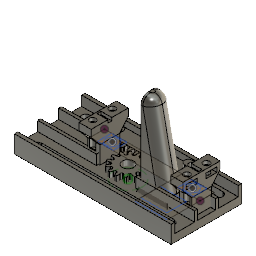
RP_Gripper_MK4_v10 (Autodesk Fusion 360 design; units mm, degrees)
description: Spur Gear; Module: 1.072000; Num Teeth: 14; Pressure Angle: 14.500000; Backlash: 0.15 mm
description: Spur Gear; Module: 1.020000; Num Teeth: 14; Pressure Angle: 14.500000; Backlash: 0.15 mm
Autodesk Fusion 360 part; units mm, degrees
sketch "Sketch1" plane through (0, 0, 0) normal (0, 0, 1) x (1, 0, 0) in component "Old Spur (14 teeth)"
  circle A0 centre (0, 0) radius 6.1668
  circle A1 centre (0, 0) radius 1.6
extrude "Extrude1" add sketch "Sketch1" along normal blind 6.5 makes body 1 in component "Old Spur (14 teeth)"
sketch "Sketch2" plane through (0, 0, 0) normal (0, 0, 1) x (1, 0, 0) in component "Old Spur (14 teeth)"
  spline S0 degree 5 poles (7.2189, -0.8174) (7.2227, -0.8178) (7.2303, -0.8185) (7.2417, -0.8194) (7.257, -0.8199) (7.2761, -0.8197) (7.2953, -0.819) (7.3145, -0.8178) (7.3337, -0.8165) (7.353, -0.815) (7.3723, -0.8134) (7.3915, -0.8117) (7.4108, -0.8096) (7.4302, -0.8073) (7.4495, -0.8047) (7.4688, -0.8019) (7.4882, -0.7988) (7.5075, -0.7955) (7.5269, -0.7921) (7.5463, -0.7884) (7.5657, -0.7847) (7.585, -0.7807) (7.6044, -0.7766) (7.6238, -0.7723) (7.6432, -0.7679) (7.6626, -0.7632) (7.682, -0.7584) (7.7014, -0.7534) (7.7208, -0.7483) (7.7402, -0.743) (7.7596, -0.7376) (7.779, -0.7321) (7.7984, -0.7264) (7.8177, -0.7205) (7.8371, -0.7145) (7.8565, -0.7084) (7.8759, -0.7021) (7.8953, -0.6956) (7.9146, -0.6891) (7.934, -0.6824) (7.9533, -0.6756) (7.9727, -0.6686) (7.992, -0.6615) (8.0114, -0.6543) (8.0307, -0.6469) (8.05, -0.6394) (8.0693, -0.6318) (8.0886, -0.6241) (8.1079, -0.6162) (8.1272, -0.6082) (8.1465, -0.6001) (8.1657, -0.5919) (8.185, -0.5835) (8.2042, -0.575) (8.2234, -0.5664) (8.2427, -0.5577) (8.2619, -0.5489) (8.281, -0.5399) (8.3002, -0.5309) (8.3194, -0.5217) (8.3385, -0.5124) (8.3577, -0.5029) (8.3768, -0.4934) (8.3959, -0.4837) (8.415, -0.474) (8.434, -0.4641) (8.4531, -0.4541) (8.4721, -0.444) (8.4911, -0.4338) (8.5101, -0.4235) (8.5291, -0.413) (8.5443, -0.4046) (8.5557, -0.3982) (8.5633, -0.394) (8.567, -0.3918) knots 0 0 0 0 0 0 0.01428571 0.02857143 0.04285714 0.05714286 0.07142857 0.08571429 0.1 0.11428571 0.12857143 0.14285714 0.15714286 0.17142857 0.18571429 0.2 0.21428571 0.22857143 0.24285714 0.25714286 0.27142857 0.28571429 0.3 0.31428571 0.32857143 0.34285714 0.35714286 0.37142857 0.38571429 0.4 0.41428571 0.42857143 0.44285714 0.45714286 0.47142857 0.48571429 0.5 0.51428571 0.52857143 0.54285714 0.55714286 0.57142857 0.58571429 0.6 0.61428571 0.62857143 0.64285714 0.65714286 0.67142857 0.68571429 0.7 0.71428571 0.72857143 0.74285714 0.75714286 0.77142857 0.78571429 0.8 0.81428571 0.82857143 0.84285714 0.85714286 0.87142857 0.88571429 0.9 0.91428571 0.92857143 0.94285714 0.95714286 0.97142857 0.98571429 1 1 1 1 1 1
  spline S1 degree 5 poles (7.2189, 0.8174) (7.2227, 0.8178) (7.2303, 0.8185) (7.2417, 0.8194) (7.257, 0.8199) (7.2761, 0.8197) (7.2953, 0.819) (7.3145, 0.8178) (7.3337, 0.8165) (7.353, 0.815) (7.3723, 0.8134) (7.3915, 0.8117) (7.4108, 0.8096) (7.4302, 0.8073) (7.4495, 0.8047) (7.4688, 0.8019) (7.4882, 0.7988) (7.5075, 0.7955) (7.5269, 0.7921) (7.5463, 0.7884) (7.5657, 0.7847) (7.585, 0.7807) (7.6044, 0.7766) (7.6238, 0.7723) (7.6432, 0.7679) (7.6626, 0.7632) (7.682, 0.7584) (7.7014, 0.7534) (7.7208, 0.7483) (7.7402, 0.743) (7.7596, 0.7376) (7.779, 0.7321) (7.7984, 0.7264) (7.8177, 0.7205) (7.8371, 0.7145) (7.8565, 0.7084) (7.8759, 0.7021) (7.8953, 0.6956) (7.9146, 0.6891) (7.934, 0.6824) (7.9533, 0.6756) (7.9727, 0.6686) (7.992, 0.6615) (8.0114, 0.6543) (8.0307, 0.6469) (8.05, 0.6394) (8.0693, 0.6318) (8.0886, 0.6241) (8.1079, 0.6162) (8.1272, 0.6082) (8.1465, 0.6001) (8.1657, 0.5919) (8.185, 0.5835) (8.2042, 0.575) (8.2234, 0.5664) (8.2427, 0.5577) (8.2619, 0.5489) (8.281, 0.5399) (8.3002, 0.5309) (8.3194, 0.5217) (8.3385, 0.5124) (8.3577, 0.5029) (8.3768, 0.4934) (8.3959, 0.4837) (8.415, 0.474) (8.434, 0.4641) (8.4531, 0.4541) (8.4721, 0.444) (8.4911, 0.4338) (8.5101, 0.4235) (8.5291, 0.413) (8.5443, 0.4046) (8.5557, 0.3982) (8.5633, 0.394) (8.567, 0.3918) knots 0 0 0 0 0 0 0.01428571 0.02857143 0.04285714 0.05714286 0.07142857 0.08571429 0.1 0.11428571 0.12857143 0.14285714 0.15714286 0.17142857 0.18571429 0.2 0.21428571 0.22857143 0.24285714 0.25714286 0.27142857 0.28571429 0.3 0.31428571 0.32857143 0.34285714 0.35714286 0.37142857 0.38571429 0.4 0.41428571 0.42857143 0.44285714 0.45714286 0.47142857 0.48571429 0.5 0.51428571 0.52857143 0.54285714 0.55714286 0.57142857 0.58571429 0.6 0.61428571 0.62857143 0.64285714 0.65714286 0.67142857 0.68571429 0.7 0.71428571 0.72857143 0.74285714 0.75714286 0.77142857 0.78571429 0.8 0.81428571 0.82857143 0.84285714 0.85714286 0.87142857 0.88571429 0.9 0.91428571 0.92857143 0.94285714 0.95714286 0.97142857 0.98571429 1 1 1 1 1 1
  arc A0 (8.567, -0.3918) -> (8.567, 0.3918) centre (0, 0) ccw
  line L0 (6.1177, -0.6938) -> (7.2189, -0.8174)
  line L1 (6.1177, 0.6938) -> (7.2189, 0.8174)
  line L2 (6.1177, -0.6938) -> (6.1177, 0.6938)
  point P0 (7.313, -0.8179)
  point P1 (7.4081, -0.8099)
  point P2 (7.5038, -0.7961)
  point P3 (7.5999, -0.7776)
  point P4 (7.6963, -0.7547)
  point P5 (7.7929, -0.7279)
  point P6 (7.8897, -0.6975)
  point P7 (7.9866, -0.6635)
  point P8 (8.0836, -0.6261)
  point P9 (8.1805, -0.5854)
  point P10 (8.2774, -0.5416)
  point P11 (8.3741, -0.4947)
  point P12 (8.4707, -0.4448)
  point P13 (7.313, 0.8179)
  point P14 (7.4081, 0.8099)
  point P15 (7.5038, 0.7961)
  point P16 (7.5999, 0.7776)
  point P17 (7.6963, 0.7547)
  point P18 (7.7929, 0.7279)
  point P19 (7.8897, 0.6975)
  point P20 (7.9866, 0.6635)
  point P21 (8.0836, 0.6261)
  point P22 (8.1805, 0.5854)
  point P23 (8.2774, 0.5416)
  point P24 (8.3741, 0.4947)
  point P25 (8.4707, 0.4448)
extrude "Extrude2" add sketch "Sketch2" along normal blind 6.5 bodies 1 in component "Old Spur (14 teeth)"
fillet "Fillet1" radius 0.6 2 edges at (6.1275, -0.6949, 3.25) (6.1275, 0.6949, 3.25) on bodies 1 in component "Old Spur (14 teeth)"
pattern_circular "C-Pattern1" count 14 over 360 about axis through (0, 0, 0) along (0, 0, 1) of "Extrude2", "Fillet1" in component "Old Spur (14 teeth)"
sketch "Sketch3" plane through (0, 0, 0) normal (0, 0, 1) x (1, 0, 0) in component "Old Spur (14 teeth)"
  circle A0 centre (0, 0) radius 7.504 construction
sketch "Sketch1 (2)" plane through (0, 0, 0) normal (0, 0, 1) x (1, 0, 0) in component "Rack"
  line L0 (-30, 8.75) -> (30, 8.75)
  line L1 (30, 8.75) -> (30, 12.75)
  line L2 (30, 12.75) -> (-30, 12.75)
  line L3 (-30, 12.75) -> (-30, 8.75)
  line L4 (0.1675, 6.2955) -> (-0.167, 6.2955)
  line L5 (-0.6525, 6.781) -> (-0.6525, 7.2573)
  line L6 (-0.6525, 9.4955) -> (0.6525, 9.4955)
  line L7 (0.6525, 9.4955) -> (0.6525, 6.7805)
  line L8 (0.6525, 6.2955) -> (-0.6525, 9.4955) construction
  line L9 (-0.6525, 6.2955) -> (0.6525, 9.4955) construction
  arc A0 (-0.6525, 6.781) -> (-0.167, 6.2955) centre (-0.167, 6.781) ccw
  arc A1 (0.1675, 6.2955) -> (0.6525, 6.7805) centre (0.1675, 6.7805) ccw
  arc A2 (-0.6724, 7.5148) -> (-1.0506, 8.75) centre (-5.1412, 6.8218) ccw
  arc A3 (-0.6525, 7.2573) -> (-0.6724, 7.5148) centre (-2.3332, 7.2573) ccw
  line L10 (0, 10) -> (0, 5.7453) construction
  arc A4 (1.0506, 8.75) -> (0.6724, 7.5148) centre (5.1412, 6.8218) ccw
  arc A5 (0.6724, 7.5148) -> (0.6525, 7.2573) centre (2.3332, 7.2573) ccw
  point P0 (0, 7.8955)
  dimension "d8" = 3.2
  dimension "d9" = 1.305
  dimension "d10" = 0.4855
  dimension "d11" = 0.485
  dimension "d12" = 1.6807
  constraint horizontal L0
  constraint vertical L1
  constraint horizontal L2
  constraint vertical L3
  constraint perpendicular L4 L5
  constraint parallel L4 L6
  constraint parallel L5 L7
  constraint horizontal L4
  constraint coincident L8 P0
  constraint coincident L9 P0
  constraint coincident L9.start L4
  constraint coincident L9.start L5
  constraint tangent L4 A0
  constraint tangent L5 A0
  constraint tangent L7 A1
  constraint tangent L4 A1
  constraint coincident L0 A2.end
  constraint coincident L6.start L5
  constraint tangent L5 A3
  constraint tangent A2 A3
  constraint perpendicular L6 L10
  constraint symmetric A2.end L10 A4.start
  constraint symmetric A2 L10 A4
  constraint symmetric L5.end L10 A5.end
  constraint symmetric A2.start L10 A4.end
  constraint symmetric A3 L10 A5
  measures "d8" distance of L9.start L6.start
  measures "d9" distance of L6.start L6.end
  measures "d10" radius of A0
  measures "d11" radius of A1
  measures "d12" radius of A3
copy_body "CopyPasteBodies1" bodies 1 makes body 2 in component "Old Spur (14 teeth)"
move_body "Move1" bodies 2 to x (0.975535, 0.219846, 0) y (-0.219846, 0.975535, 0) z (0, 0, 1) at (0, 0, 0) in component "Old Spur (14 teeth)"
extrude "Extrude1'" add sketch "Sketch1 (2)" along normal blind 6 separate body contours L0 L4 L5 L7 A0 A1 A2 A3 | L0 L7 A4 A5 makes body 3 in component "Rack"
move_body "Move2" bodies 2 to x (1, 0, 0) y (0, 1, 0) z (0, 0, 1) at (-1.6805, 0, 0) in component "Old Spur (14 teeth)"
copy_body "CopyPasteBodies1'" bodies 3 makes body 4 in component "Rack"
move_body "Move1'" bodies 4 to x (1, 0, 0) y (0, 1, 0) z (0, 0, 1) at (-3.31, 0, 0) in component "Rack"
copy_body "CopyPasteBodies2" bodies 4 makes body 5 in component "Rack"
move_body "Move2'" bodies 5 to x (1, 0, 0) y (0, 1, 0) z (0, 0, 1) at (-3.31, 0, 0) in component "Rack"
copy_body "CopyPasteBodies3" bodies 5 makes body 6 in component "Rack"
move_body "Move3" bodies 6 to x (1, 0, 0) y (0, 1, 0) z (0, 0, 1) at (-3.31, 0, 0) in component "Rack"
copy_body "CopyPasteBodies4" bodies 6 makes body 7 in component "Rack"
move_body "Move4" bodies 7 to x (1, 0, 0) y (0, 1, 0) z (0, 0, 1) at (-3.31, 0, 0) in component "Rack"
copy_body "CopyPasteBodies5" bodies 7 makes body 8 in component "Rack"
move_body "Move5" bodies 8 to x (1, 0, 0) y (0, 1, 0) z (0, 0, 1) at (-3.31, 0, 0) in component "Rack"
copy_body "CopyPasteBodies6" bodies 8 makes body 9 in component "Rack"
move_body "Move6" bodies 9 to x (1, 0, 0) y (0, 1, 0) z (0, 0, 1) at (-3.31, 0, 0) in component "Rack"
copy_body "CopyPasteBodies7" bodies 9 makes body 10 in component "Rack"
move_body "Move7" bodies 10 to x (1, 0, 0) y (0, 1, 0) z (0, 0, 1) at (-3.31, 0, 0) in component "Rack"
copy_body "CopyPasteBodies8" bodies 10 makes body 11 in component "Rack"
move_body "Move8" bodies 11 to x (1, 0, 0) y (0, 1, 0) z (0, 0, 1) at (-3.31, 0, 0) in component "Rack"
copy_body "CopyPasteBodies9" bodies 3 makes body 12 in component "Rack"
move_body "Move9" bodies 12 to x (1, 0, 0) y (0, 1, 0) z (0, 0, 1) at (3.31, 0, 0) in component "Rack"
copy_body "CopyPasteBodies10" bodies 12 makes body 13 in component "Rack"
move_body "Move10" bodies 13 to x (1, 0, 0) y (0, 1, 0) z (0, 0, 1) at (3.31, 0, 0) in component "Rack"
copy_body "CopyPasteBodies11" bodies 13 makes body 14 in component "Rack"
move_body "Move11" bodies 14 to x (1, 0, 0) y (0, 1, 0) z (0, 0, 1) at (3.31, 0, 0) in component "Rack"
copy_body "CopyPasteBodies12" bodies 14 makes body 15 in component "Rack"
move_body "Move12" bodies 15 to x (1, 0, 0) y (0, 1, 0) z (0, 0, 1) at (3.31, 0, 0) in component "Rack"
copy_body "CopyPasteBodies13" bodies 15 makes body 16 in component "Rack"
move_body "Move13" bodies 16 to x (1, 0, 0) y (0, 1, 0) z (0, 0, 1) at (3.31, 0, 0) in component "Rack"
copy_body "CopyPasteBodies14" bodies 16 makes body 17 in component "Rack"
move_body "Move14" bodies 17 to x (1, 0, 0) y (0, 1, 0) z (0, 0, 1) at (3.31, 0, 0) in component "Rack"
copy_body "CopyPasteBodies15" bodies 17 makes body 18 in component "Rack"
move_body "Move15" bodies 18 to x (1, 0, 0) y (0, 1, 0) z (0, 0, 1) at (3.31, 0, 0) in component "Rack"
copy_body "CopyPasteBodies16" bodies 18 makes body 19 in component "Rack"
move_body "Move16" bodies 19 to x (1, 0, 0) y (0, 1, 0) z (0, 0, 1) at (3.31, 0, 0) in component "Rack"
sketch "Sketch2 (2)" plane through (0, 0, 0) normal (0, 0, 1) x (1, 0, 0) in component "Rack"
  line L0 (28, 16) -> (-28, 16)
  line L1 (-28, 16) -> (-28, 8.75)
  line L2 (-28, 8.75) -> (28, 8.75)
  line L3 (28, 8.75) -> (28, 16)
  dimension "d15" = 56
  dimension "d16" = 7.25
  constraint horizontal L0
  constraint vertical L1
  constraint horizontal L2
  constraint vertical L3
  measures "d15" distance of L0.start L0.end
  measures "d16" distance of L0.start L2.end
extrude "Extrude2'" add sketch "Sketch2 (2)" along normal blind 6 separate body makes body 20 in component "Rack"
sketch "Sketch1 (3)" plane through (0, 0, 0) normal (0, 0, 1) x (1, 0, 0) in component "Base"
  line L0 (40, 18) -> (-40, 18)
  line L1 (-40, 18) -> (-40, -18)
  line L2 (-40, -18) -> (40, -18)
  line L3 (40, -18) -> (40, 18)
  line L4 (-40, 18) -> (40, 18)
  line L5 (40, 18) -> (40, 16.2)
  line L6 (40, 16.2) -> (-40, 16.2)
  line L7 (-40, 16.2) -> (-40, 18)
  line L8 (40, 4.6) -> (10, 4.6)
  line L9 (10, 4.6) -> (10, 6.1)
  line L10 (10, 6.1) -> (40, 6.1)
  line L11 (40, 6.1) -> (40, 4.6)
  line L12 (-40, 4.6) -> (-10, 4.6)
  line L13 (-10, 4.6) -> (-10, 6.1)
  line L14 (-10, 6.1) -> (-40, 6.1)
  line L15 (-40, 6.1) -> (-40, 4.6)
  line L16 (-40, -18) -> (40, -18)
  line L17 (40, -18) -> (40, -16.2)
  line L18 (40, -16.2) -> (-40, -16.2)
  line L19 (-40, -16.2) -> (-40, -18)
  line L20 (40, -4.6) -> (10, -4.6)
  line L21 (10, -4.6) -> (10, -6.1)
  line L22 (10, -6.1) -> (40, -6.1)
  line L23 (40, -6.1) -> (40, -4.6)
  line L24 (-40, -4.6) -> (-10, -4.6)
  line L25 (-10, -4.6) -> (-10, -6.1)
  line L26 (-10, -6.1) -> (-40, -6.1)
  line L27 (-40, -6.1) -> (-40, -4.6)
  line L28 (45.5245, 12.375) -> (-50, 12.375) construction
  line L29 (33.9, 14.475) -> (-33.9, 14.475)
  line L30 (-36, 12.375) -> (-36, 12.375)
  line L31 (-33.9, 10.275) -> (33.9, 10.275)
  line L32 (36, 12.375) -> (36, 12.375)
  arc A0 (33.9, 10.275) -> (36, 12.375) centre (33.9, 12.375) ccw
  arc A1 (36, 12.375) -> (33.9, 14.475) centre (33.9, 12.375) ccw
  arc A2 (-33.9, 14.475) -> (-36, 12.375) centre (-33.9, 12.375) ccw
  arc A3 (-36, 12.375) -> (-33.9, 10.275) centre (-33.9, 12.375) ccw
  line L33 (45, 0) -> (-44, 0) construction
  arc A4 (-36, -12.375) -> (-33.9, -14.475) centre (-33.9, -12.375) ccw
  arc A5 (-33.9, -10.275) -> (-36, -12.375) centre (-33.9, -12.375) ccw
  line L34 (-33.9, -10.275) -> (33.9, -10.275)
  line L35 (33.9, -14.475) -> (-33.9, -14.475)
  arc A6 (36, -12.375) -> (33.9, -10.275) centre (33.9, -12.375) ccw
  arc A7 (33.9, -14.475) -> (36, -12.375) centre (33.9, -12.375) ccw
  point P0 (36, 14.475)
  point P1 (36, 10.275)
  dimension "d19" = 1.8
  dimension "d20" = 80
  dimension "d21" = 30
  dimension "d22" = 1.5
  dimension "d23" = 10.1
  dimension "d24" = 30
  dimension "d25" = 1.5
  dimension "d26" = 10.1
  dimension "d27" = 80
  dimension "d28" = 1.8
  dimension "d29" = 30
  dimension "d30" = 1.5
  dimension "d31" = 10.1
  dimension "d32" = 30
  dimension "d33" = 1.5
  dimension "d34" = 10.1
  dimension "d35" = 4.2
  dimension "d36" = 2.1
  dimension "d37" = 2.1
  dimension "d38" = 2.1
  dimension "d39" = 2.1
  dimension "d40" = 2.1
  constraint horizontal L0
  constraint vertical L1
  constraint horizontal L2
  constraint vertical L3
  constraint horizontal L4
  constraint vertical L5
  constraint horizontal L6
  constraint vertical L7
  constraint horizontal L8
  constraint vertical L9
  constraint horizontal L10
  constraint vertical L11
  constraint coincident L3 L8.start
  constraint horizontal L12
  constraint vertical L13
  constraint horizontal L14
  constraint vertical L15
  constraint coincident L1 L12.start
  constraint horizontal L16
  constraint vertical L17
  constraint horizontal L18
  constraint vertical L19
  constraint horizontal L20
  constraint vertical L21
  constraint horizontal L22
  constraint vertical L23
  constraint coincident L3 L20.start
  constraint horizontal L24
  constraint vertical L25
  constraint horizontal L26
  constraint vertical L27
  constraint coincident L1 L24.start
  constraint perpendicular L3 L28
  constraint horizontal L29
  constraint horizontal L31
  constraint coincident P1 L31
  constraint tangent L31 A0
  constraint coincident P0 L29
  constraint coincident P0 L32
  constraint tangent L29 A1
  constraint tangent L29 A2
  constraint tangent L31 A3
  constraint perpendicular L3 L33
  constraint symmetric L31.end L33 L34.end
  constraint symmetric L32.start L33 A6.start
  constraint symmetric A0 L33 A6
  constraint symmetric L29.start L33 L35.start
  constraint symmetric A1 L33 A7
  constraint symmetric L29.end L33 A4.end
  constraint symmetric L30.start L33 A4.start
  constraint symmetric A2 L33 A4
  constraint symmetric L31.start L33 A5.start
  constraint symmetric A3 L33 A5
  measures "d19" distance of L0.end L6.end
  measures "d20" distance of L0.end L0.start
  measures "d21" distance of L8.start L8.end
  measures "d22" distance of L8.start L10.end
  measures "d23" distance of L6 L10
  measures "d24" distance of L12.start L12.end
  measures "d25" distance of L12.start L14.end
  measures "d26" distance of L6 L14
  measures "d27" distance of L1.end L2.end
  measures "d28" distance of L1.end L18.end
  measures "d29" distance of L20.start L20.end
  measures "d30" distance of L20.start L22.end
  measures "d31" distance of L18 L22
  measures "d32" distance of L24.start L24.end
  measures "d33" distance of L24.start L26.end
  measures "d34" distance of L18 L26
  measures "d35" distance of P0 P1
  measures "d36" distance of L28 L29
  measures "d37" radius of A0
  measures "d38" radius of A1
  measures "d39" radius of A2
  measures "d40" radius of A3
extrude "Extrude1''" add sketch "Sketch1 (3)" along normal blind 4 separate body makes body 21 in component "Base"
extrude "Extrude2''" add sketch "Sketch1 (3)" along normal blind 9 contours L0 L1 L3 L4 L5 L6 L7 | L3 L8 L9 L10 L11 | L1 L12 L13 L14 L15 | L3 L20 L21 L22 L23 | L1 L24 L25 L26 L27 | L1 L2 L3 L16 L17 L18 L19 bodies 21 in component "Base"
box "BoxPrimitive1" add length 10 width 6.25 height 9 placed x (0, -1, 0) y (1, 0, 0) z (0, 0, 1) at (-15.25, 5, 4) separate body makes body 22 in component "Base"
box "BoxPrimitive2" add length 19 width 6.25 height 9 placed x (0, -1, 0) y (1, 0, 0) z (0, 0, 1) at (-15.25, 8.9473, 13) separate body makes body 23 in component "Base"
move_body "Move1''" bodies 23 to x (1, 0, 0) y (0, 1, 0) z (0, 0, 1) at (0, 0, 15.6817) in component "Base"
move_body "Align1" bodies 23 to x (1, 0, 0) y (0, 1, 0) z (0, 0, 1) at (0, 0.5527, -15.6817) in component "Base"
chamfer "Chamfer1" distance 4.5 angle 50 2 edges at (-12.125, -9.5, 13) (-12.125, 9.5, 13) measured on face at (-11.0833, 3.1667, 13) measured on face at (-11.0833, 3.1667, 13) on bodies 23 in component "Base"
sketch "Sketch4" plane through (0, 0, 22) normal (0, 0, 1) x (-1, 0, 0) in component "Base"
  line L0 (15.25, 9.5) -> (9, 9.5)
  line L1 (9, 9.5) -> (9, -9.5)
  line L2 (9, -9.5) -> (15.25, -9.5)
  line L3 (15.25, -9.5) -> (15.25, 9.5)
  circle A0 centre (12.75, -5) radius 1.6
  circle A1 centre (12.75, 5) radius 1.6
  line L4 (9, 1) -> (14.5, 1)
  line L5 (14.5, 1) -> (14.5, -1)
  line L6 (14.5, -1) -> (9, -1)
  line L7 (9, -1) -> (9, 1)
  dimension "d57" = 3.2
  dimension "d58" = 4.5
  dimension "d59" = 2.5
  dimension "d60" = 3.2
  dimension "d61" = 2.5
  dimension "d62" = 10
  dimension "d63" = 5.5
  dimension "d64" = 2
  constraint horizontal L4
  constraint vertical L5
  constraint horizontal L6
  constraint vertical L7
  constraint coincident L1 L4.start
  measures "d57" diameter of A0
  measures "d58" distance of L2 A0.centre
  measures "d59" distance of L3 A0.centre
  measures "d60" diameter of A1
  measures "d61" distance of L3 A1.centre
  measures "d62" vertical distance of A0.centre A1.centre
  measures "d63" distance of L4.start L4.end
  measures "d64" distance of L4.start L6.end
extrude "Extrude3" cut sketch "Sketch4" against normal blind 13 contours A0 | A1 bodies 22 23 in component "Base"
extrude "Extrude4" cut sketch "Sketch4" against normal blind 1.5 contours L1 L4 L5 L6 L7 bodies 23 in component "Base"
sketch "Sketch5" plane through (-15.25, 0, 0) normal (-1, 0, 0) x (0, -1, 0) in component "Base"
  line L0 (-9.5, 18.3629) -> (-5, 13)
  line L1 (-5, 13) -> (5, 13)
  line L2 (5, 13) -> (9.5, 18.3629)
  line L3 (9.5, 18.3629) -> (9.5, 22)
  line L4 (9.5, 22) -> (-9.5, 22)
  line L5 (-9.5, 22) -> (-9.5, 18.3629)
  line L6 (-7.8, 20.25) -> (-2.2, 20.25)
  line L7 (-2.2, 20.25) -> (-2.2, 17.75)
  line L8 (-2.2, 17.75) -> (-7.8, 17.75)
  line L9 (-7.8, 17.75) -> (-7.8, 20.25)
  line L10 (-3.4, 22) -> (-6.6, 22)
  line L11 (0, 23) -> (0, 12) construction
  line L12 (7.8, 17.75) -> (7.8, 20.25)
  line L13 (7.8, 20.25) -> (2.2, 20.25)
  line L14 (2.2, 20.25) -> (2.2, 17.75)
  line L15 (2.2, 17.75) -> (7.8, 17.75)
  dimension "d69" = 5.6
  dimension "d70" = 2.5
  dimension "d71" = 1.7
  dimension "d72" = 1.75
  constraint horizontal L6
  constraint vertical L7
  constraint horizontal L8
  constraint vertical L9
  constraint perpendicular L1 L11
  constraint symmetric L6.start L11 L12.end
  constraint symmetric L6.end L11 L13.end
  constraint symmetric L7.end L11 L14.end
  constraint symmetric L8.end L11 L12.start
  measures "d69" distance of L6.start L6.end
  measures "d70" distance of L6.start L8.end
  measures "d71" distance of L5 L9
  measures "d72" distance of L6 L10
extrude "Extrude5" cut sketch "Sketch5" against normal blind 5.6 contours L6 L7 L8 L9 | L12 L13 L14 L15 bodies 23 in component "Base"
copy_body "CopyPasteBodies1''" bodies 22 23 makes body 24 makes body 25 in component "Base"
move_body "Move2''" bodies 24 25 to x (1, 0, 0) y (0, 1, 0) z (0, 0, 1) at (45, 0, 0) in component "Base"
move_body "Move3'" bodies 25 24 to x (-1, 0, 0) y (0, -1, 0) z (0, 0, 1) at (66.5, 0, 0) in component "Base"
move_body "Move4'" bodies 22 23 to x (1, 0, 0) y (0, 1, 0) z (0, 0, 1) at (-4, 0, 0) in component "Base"
move_body "Move5'" bodies 25 24 to x (1, 0, 0) y (0, 1, 0) z (0, 0, 1) at (-3, 0, 0) in component "Base"
box "BoxPrimitive1'" add length 4 width 48.8 height 4.3 placed x (0, -1, 0) y (1, 0, 0) z (0, 0, 1) at (-28, 16, 6) separate body makes body 26 in component "Rack"
move_body "Move17" bodies 26 to x (1, 0, 0) y (0, 1, 0) z (0, 0, 1) at (3.61, 0, 0) in component "Rack"
move_body "Move18" bodies 26 to x (1, 0, 0) y (0, 1, 0) z (0, 0, 1) at (0, -1.625, 0) in component "Rack"
ref_plane "WorkPlane1" through (-16.39, 12.375, 8.15) normal (-1, 0, 0) x (0, 0, -1) in component "Rack"
split "Split1" by plane through (-16.39, 12.375, 8.15) normal (-1, 0, 0) bodies 26 makes body 27 at (-21.7233, 14.375, 7.4333) in component "Rack"
ref_plane "WorkPlane2" through (16.41, 12.375, 8.15) normal (1, 0, 0) x (0, 0, 1) in component "Rack"
split "Split2" by plane through (16.41, 12.375, 8.15) normal (1, 0, 0) bodies 26 makes body 28 at (19.0767, 14.375, 7.4333) in component "Rack"
delete_body "RemoveBody1" bodies 26 in component "Rack"
sketch "Sketch4 (2)" plane through (0, 0, 10.3) normal (0, 0, 1) x (-1, 0, 0) in component "Rack"
  line L0 (16.39, -10.375) -> (16.39, -14.375)
  line L1 (16.39, -14.375) -> (24.39, -14.375)
  line L2 (24.39, -14.375) -> (24.39, -10.375)
  line L3 (24.39, -10.375) -> (16.39, -10.375)
  circle A0 centre (20.39, -12.375) radius 1.65
  dimension "d83" = 3.3
  dimension "d84" = 2
  dimension "d85" = 4
  measures "d83" diameter of A0
  measures "d84" distance of L1 A0.centre
  measures "d85" distance of L2 A0.centre
sketch "Sketch5 (2)" plane through (0, 0, 10.3) normal (0, 0, 1) x (-1, 0, 0) in component "Rack"
  line L0 (-16.41, -14.375) -> (-16.41, -10.375)
  line L1 (-16.41, -10.375) -> (-24.41, -10.375)
  line L2 (-24.41, -10.375) -> (-24.41, -14.375)
  line L3 (-24.41, -14.375) -> (-16.41, -14.375)
  circle A0 centre (-20.41, -12.375) radius 1.65
  dimension "d86" = 3.3
  dimension "d87" = 4
  dimension "d88" = 2
  measures "d86" diameter of A0
  measures "d87" distance of L2 A0.centre
  measures "d88" distance of L3 A0.centre
fillet "Fillet2" radius 2 4 edges at (24.41, 10.375, 8.15) (16.41, 10.375, 8.15) (24.41, 14.375, 8.15) (16.41, 14.375, 8.15) on bodies 28 in component "Rack"
fillet "Fillet3" radius 2 4 edges at (-16.39, 14.375, 8.15) (-24.39, 14.375, 8.15) (-24.39, 10.375, 8.15) (-16.39, 10.375, 8.15) on bodies 27 in component "Rack"
extrude "Extrude3'" cut sketch "Sketch4 (2)" against normal blind 21.743 contours A0 bodies 20 27 in component "Rack"
extrude "Extrude4'" cut sketch "Sketch5 (2)" against normal blind 14.123 contours A0 bodies 20 28 in component "Rack"
sketch "Sketch6" plane through (0, 0, 0) normal (0, 0, -1) x (1, 0, 0) in component "Rack"
  circle A0 centre (20.41, -12.375) radius 1.65
  circle A1 centre (-20.39, -12.375) radius 1.65
  line L0 (28, -16) -> (28, -8.75)
  line L1 (28, -8.75) -> (-28, -8.75)
  line L2 (-28, -8.75) -> (-28, -16)
  line L3 (-28, -16) -> (28, -16)
  circle A2 centre (-20.39, -12.375) radius 3.1
  circle A3 centre (20.41, -12.375) radius 3.1
  dimension "d95" = 6.2
  dimension "d96" = 6.2
  constraint concentric A1 A2
  constraint concentric A0 A3
  measures "d95" diameter of A2
  measures "d96" diameter of A3
extrude "Extrude5'" cut sketch "Sketch6" against normal blind 2.8 contours A2 | A3 bodies 20 in component "Rack"
sketch "Sketch1 (4)" plane through (0, 0, 0) normal (0, 0, 1) x (1, 0, 0) in component "Jaw"
  line L0 (-28, 16) -> (28, 16)
  line L1 (28, 16) -> (28, 8.75)
  line L2 (28, 8.75) -> (-28, 8.75)
  line L3 (-28, 8.75) -> (-28, 16)
  line L4 (11.5, 16) -> (28, 16)
  line L5 (28, 16) -> (28, -8)
  line L6 (28, -8) -> (11.5, -8)
  line L7 (11.5, -8) -> (11.5, 16)
  line L8 (11.5, -5) -> (24.8331, -5)
  line L9 (24.8331, -5) -> (24.8331, 5)
  line L10 (24.8331, 5) -> (11.5, 5)
  line L11 (11.5, 5) -> (11.5, -5)
  circle A0 centre (20.4076, 12.375) radius 1.6
  circle A1 centre (-20.3901, 12.3735) radius 1.6
  line L12 (-16.3901, 8.8735) -> (-24.3901, 8.8735)
  line L13 (-24.3901, 8.8735) -> (-24.3901, 15.8735)
  line L14 (-24.3901, 15.8735) -> (-16.3901, 15.8735)
  line L15 (-16.3901, 15.8735) -> (-16.3901, 8.8735)
  line L16 (-16.3901, 8.8735) -> (-24.3901, 15.8735) construction
  line L17 (-24.3901, 8.8735) -> (-16.3901, 15.8735) construction
  line L18 (-18.7157, 9.4735) -> (-17.0414, 12.3735)
  line L19 (-17.0414, 12.3735) -> (-18.7157, 15.2735)
  line L20 (-18.7157, 15.2735) -> (-22.0644, 15.2735)
  line L21 (-22.0644, 15.2735) -> (-23.7387, 12.3735)
  line L22 (-23.7387, 12.3735) -> (-22.0644, 9.4735)
  line L23 (-22.0644, 9.4735) -> (-18.7157, 9.4735)
  line L24 (24.4076, 8.875) -> (16.4076, 8.875)
  line L25 (16.4076, 8.875) -> (16.4076, 15.875)
  line L26 (16.4076, 15.875) -> (24.4076, 15.875)
  line L27 (24.4076, 15.875) -> (24.4076, 8.875)
  line L28 (24.4076, 8.875) -> (16.4076, 15.875) construction
  line L29 (16.4076, 8.875) -> (24.4076, 15.875) construction
  line L30 (22.0819, 9.475) -> (23.7562, 12.375)
  line L31 (23.7562, 12.375) -> (22.0819, 15.275)
  line L32 (22.0819, 15.275) -> (18.7333, 15.275)
  line L33 (18.7333, 15.275) -> (17.0589, 12.375)
  line L34 (17.0589, 12.375) -> (18.7333, 9.475)
  line L35 (18.7333, 9.475) -> (22.0819, 9.475)
  point P0 (-28, 16)
  point P1 (28, 8.75)
  point P2 (-20.3901, 12.3735)
  point P3 (-20.3901, 12.3735)
  point P4 (20.4076, 12.375)
  point P5 (20.4076, 12.375)
  dimension "d99" = 3.2
  dimension "d100" = 3.2
  dimension "d115" = 8
  dimension "d116" = 7
  dimension "d117" = 8
  dimension "d118" = 7
  dimension "d153" = 39.5
  dimension "d154" = 16.5
  constraint horizontal L0
  constraint vertical L1
  constraint horizontal L2
  constraint vertical L3
  constraint coincident P1 L1.end
  constraint coincident P0 L0.start
  constraint horizontal L4
  constraint vertical L5
  constraint horizontal L6
  constraint vertical L7
  constraint coincident L0 L4.start
  constraint horizontal L8
  constraint vertical L9
  constraint horizontal L10
  constraint vertical L11
  constraint coincident L7 L8.start
  constraint perpendicular L12 L13
  constraint parallel L12 L14
  constraint parallel L13 L15
  constraint horizontal L12
  constraint coincident L16 P3
  constraint coincident L17 P3
  constraint coincident P3 P2
  constraint perpendicular L24 L25
  constraint parallel L24 L26
  constraint parallel L25 L27
  constraint horizontal L24
  constraint coincident L28 P5
  constraint coincident L29 P5
  constraint coincident P5 P4
  measures "d99" diameter of A0
  measures "d100" diameter of A1
  measures "d115" distance of L13.end L14.end
  measures "d116" distance of L12.end L13.end
  measures "d117" distance of L25.end L26.end
  measures "d118" distance of L24.end L25.end
  measures "d153" distance of L3 L7
  measures "d154" horizontal distance of L5.end L6.end
extrude "Extrude1'''" add sketch "Sketch1 (4)" along normal blind 3 separate body contours L0 L2 L3 L7 | L0 L1 L2 L4 L5 L7 | L2 L5 L6 L7 L8 L9 L10 | L7 L8 L9 L10 L11 | L12 L13 L14 L15 | L18 L19 L20 L21 L22 L23 | L24 L25 L26 L27 | L30 L31 L32 L33 L34 L35 makes body 29 in component "Jaw"
extrude "Extrude2'''" add sketch "Sketch1 (4)" along normal blind 6 separate body contours L2 L5 L6 L7 L8 L9 L10 | L7 L8 L9 L10 L11 makes body 30 in component "Jaw"
chamfer "Chamfer1'" distance 3 angle 45 1 edges at (19.75, -8, 6) on bodies 30 in component "Jaw"
chamfer "Chamfer2" distance 3 angle 45 1 edges at (28, 1.875, 6) on bodies 30 in component "Jaw"
chamfer "Chamfer3" distance 3.75 angle 45 1 edges at (18.25, 8.75, 6) on bodies 30 in component "Jaw"
extrude "Extrude3''" add sketch "Sketch1 (4)" along normal blind 45 contours L7 L8 L9 L10 L11 bodies 29 30 in component "Jaw"
chamfer "Chamfer4" distance 8 distance2 39 1 edges at (24.8331, 0, 45) measured on face at (15.9444, -1.6667, 45) on bodies 29 in component "Jaw"
fillet "Fillet1'" radius 5 2 edges at (20.8331, -5, 25.5) (20.8331, 5, 25.5) on bodies 29 in component "Jaw"
extrude "Extrude4''" add sketch "Sketch1 (4)" along normal blind 6 separate body contours L12 L13 L14 L15 | L24 L25 L26 L27 makes body 31 at (-19.0567, 8.8735, 2) makes body 32 at (21.7409, 8.875, 2) in component "Jaw"
fillet "Fillet3'" radius 2 4 edges at (-24.3901, 8.8735, 3) (-16.3901, 8.8735, 3) (-16.3901, 15.8735, 3) (-24.3901, 15.8735, 3) on bodies 31 in component "Jaw"
fillet "Fillet4" radius 2 4 edges at (16.4076, 15.875, 3) (24.4076, 15.875, 3) (24.4076, 8.875, 3) (16.4076, 8.875, 3) on bodies 32 in component "Jaw"
fillet "Fillet5" radius 1 5 edges at (28, -8, 1.5) (11.5, -8, 1.5) (28, 16, 1.5) (-28, 16, 1.5) (-28, 8.75, 1.5) on bodies 29 in component "Jaw"
box "BoxPrimitive1''" add length 7 width 6 height 2 placed x (0, 1, 0) y (-1, 0, 0) z (0, 0, 1) at (37, -1, 0) separate body makes body 33 in component "Jaw"
chamfer "Chamfer5" distance 3 distance2 2 1 edges at (31, 2.5, 2) measured on face at (33, 1.3333, 2) on bodies 33 in component "Jaw"
move_body "Move1'''" bodies 33 to x (1, 0, 0) y (0, 1, 0) z (0, 0, 1) at (-6, 0, 0) in component "Jaw"
combine "Combine1" operation cut target body 29 tool bodies 33 in component "Jaw"
cylinder "CylinderPrimitive1" cut diameter 5.7 height -3.2 placed x (1, 0, 0) y (0, 1, 0) z (0, 0, 1) at (0, 0, 6.5) bodies 1 in component "Old Spur (14 teeth)"
cylinder "CylinderPrimitive2" cut diameter 6.2 height -2.2 placed x (0, 1, 0) y (1, 0, 0) z (0, 0, -1) at (0, 0, 0) bodies 1 in component "Old Spur (14 teeth)"
box "BoxPrimitive2'" cut length 5.25 width 1.22 height -4.2 placed x (0, 1, 0) y (-1, 0, 0) z (0, 0, 1) at (-19.78, 9.75, 10.3) bodies 27 in component "Rack"
box "BoxPrimitive3" cut length 5.2994 width 1.22 height -4.2 placed x (0, -1, 0) y (1, 0, 0) z (0, 0, 1) at (19.78, 15, 10.3) bodies 28 in component "Rack"
extrude "Extrude6" cut 1 faces at (11.3, 14.475, 1.3333) along direction (0, 1, 0) blind 0.1 on bodies 21 bodies 21 in component "Base"
extrude "Extrude7" cut 1 faces at (-11.3, -10.275, 1.3333) along direction (0, 1, 0) blind 0.1 on bodies 21 bodies 21 in component "Base"
extrude "Extrude8" cut 1 faces at (11.3, -14.475, 1.3333) along direction (0, -1, 0) blind 0.1 on bodies 21 bodies 21 in component "Base"
extrude "Extrude9" cut 1 faces at (-11.3, 10.275, 1.3333) along direction (0, -1, 0) blind 0.1 on bodies 21 bodies 21 in component "Base"
move_body "Move6'" bodies 25 24 23 22 to x (1, 0, 0) y (0, 1, 0) z (0, 0, 1) at (3.75, 0, 0) in component "Base"
fillet "Fillet6" radius 4 4 edges at (11.6145, 5, 45) (15.3381, 3.5355, 45) (15.3381, -3.5355, 45) (11.6145, -5, 45) on bodies 29 in component "Jaw"
sketch "Sketch1 (5)" plane through (0, 0, 0) normal (0, 0, 1) x (1, 0, 0) in component "Spur Gear (14 teeth) (1)"
  circle A0 centre (0, 0) radius 5.8652
  circle A1 centre (0, 0) radius 1.6
extrude "Extrude1''''" add sketch "Sketch1 (5)" along normal blind 6.5 separate body makes body 34 in component "Spur Gear (14 teeth) (1)"
sketch "Sketch2 (3)" plane through (0, 0, 0) normal (0, 0, 1) x (1, 0, 0) in component "Spur Gear (14 teeth) (1)"
  spline S0 degree 5 poles (6.8689, -0.776) (6.8725, -0.7764) (6.8797, -0.7771) (6.8906, -0.7779) (6.9051, -0.7783) (6.9233, -0.7782) (6.9416, -0.7775) (6.9598, -0.7764) (6.9781, -0.7751) (6.9965, -0.7737) (7.0148, -0.7722) (7.0331, -0.7705) (7.0515, -0.7686) (7.0699, -0.7664) (7.0882, -0.7639) (7.1066, -0.7612) (7.125, -0.7582) (7.1435, -0.7551) (7.1619, -0.7518) (7.1803, -0.7484) (7.1987, -0.7448) (7.2172, -0.7411) (7.2356, -0.7371) (7.254, -0.733) (7.2725, -0.7288) (7.2909, -0.7244) (7.3094, -0.7198) (7.3278, -0.7151) (7.3463, -0.7102) (7.3647, -0.7052) (7.3832, -0.7) (7.4016, -0.6947) (7.4201, -0.6893) (7.4385, -0.6837) (7.457, -0.678) (7.4754, -0.6721) (7.4939, -0.6662) (7.5123, -0.66) (7.5307, -0.6538) (7.5491, -0.6474) (7.5676, -0.6409) (7.586, -0.6343) (7.6044, -0.6275) (7.6228, -0.6207) (7.6412, -0.6136) (7.6595, -0.6065) (7.6779, -0.5993) (7.6963, -0.5919) (7.7146, -0.5844) (7.733, -0.5768) (7.7513, -0.5691) (7.7696, -0.5612) (7.788, -0.5533) (7.8063, -0.5452) (7.8246, -0.537) (7.8428, -0.5287) (7.8611, -0.5203) (7.8794, -0.5118) (7.8976, -0.5031) (7.9159, -0.4944) (7.9341, -0.4855) (7.9523, -0.4766) (7.9705, -0.4675) (7.9887, -0.4583) (8.0068, -0.449) (8.025, -0.4396) (8.0431, -0.4301) (8.0612, -0.4204) (8.0793, -0.4107) (8.0974, -0.4009) (8.1155, -0.391) (8.1299, -0.3829) (8.1408, -0.3769) (8.148, -0.3728) (8.1516, -0.3707) knots 0 0 0 0 0 0 0.01428571 0.02857143 0.04285714 0.05714286 0.07142857 0.08571429 0.1 0.11428571 0.12857143 0.14285714 0.15714286 0.17142857 0.18571429 0.2 0.21428571 0.22857143 0.24285714 0.25714286 0.27142857 0.28571429 0.3 0.31428571 0.32857143 0.34285714 0.35714286 0.37142857 0.38571429 0.4 0.41428571 0.42857143 0.44285714 0.45714286 0.47142857 0.48571429 0.5 0.51428571 0.52857143 0.54285714 0.55714286 0.57142857 0.58571429 0.6 0.61428571 0.62857143 0.64285714 0.65714286 0.67142857 0.68571429 0.7 0.71428571 0.72857143 0.74285714 0.75714286 0.77142857 0.78571429 0.8 0.81428571 0.82857143 0.84285714 0.85714286 0.87142857 0.88571429 0.9 0.91428571 0.92857143 0.94285714 0.95714286 0.97142857 0.98571429 1 1 1 1 1 1
  spline S1 degree 5 poles (6.8689, 0.776) (6.8725, 0.7764) (6.8797, 0.7771) (6.8906, 0.7779) (6.9051, 0.7783) (6.9233, 0.7782) (6.9416, 0.7775) (6.9598, 0.7764) (6.9781, 0.7751) (6.9965, 0.7737) (7.0148, 0.7722) (7.0331, 0.7705) (7.0515, 0.7686) (7.0699, 0.7664) (7.0882, 0.7639) (7.1066, 0.7612) (7.125, 0.7582) (7.1435, 0.7551) (7.1619, 0.7518) (7.1803, 0.7484) (7.1987, 0.7448) (7.2172, 0.7411) (7.2356, 0.7371) (7.254, 0.733) (7.2725, 0.7288) (7.2909, 0.7244) (7.3094, 0.7198) (7.3278, 0.7151) (7.3463, 0.7102) (7.3647, 0.7052) (7.3832, 0.7) (7.4016, 0.6947) (7.4201, 0.6893) (7.4385, 0.6837) (7.457, 0.678) (7.4754, 0.6721) (7.4939, 0.6662) (7.5123, 0.66) (7.5307, 0.6538) (7.5491, 0.6474) (7.5676, 0.6409) (7.586, 0.6343) (7.6044, 0.6275) (7.6228, 0.6207) (7.6412, 0.6136) (7.6595, 0.6065) (7.6779, 0.5993) (7.6963, 0.5919) (7.7146, 0.5844) (7.733, 0.5768) (7.7513, 0.5691) (7.7696, 0.5612) (7.788, 0.5533) (7.8063, 0.5452) (7.8246, 0.537) (7.8428, 0.5287) (7.8611, 0.5203) (7.8794, 0.5118) (7.8976, 0.5031) (7.9159, 0.4944) (7.9341, 0.4855) (7.9523, 0.4766) (7.9705, 0.4675) (7.9887, 0.4583) (8.0068, 0.449) (8.025, 0.4396) (8.0431, 0.4301) (8.0612, 0.4204) (8.0793, 0.4107) (8.0974, 0.4009) (8.1155, 0.391) (8.1299, 0.3829) (8.1408, 0.3769) (8.148, 0.3728) (8.1516, 0.3707) knots 0 0 0 0 0 0 0.01428571 0.02857143 0.04285714 0.05714286 0.07142857 0.08571429 0.1 0.11428571 0.12857143 0.14285714 0.15714286 0.17142857 0.18571429 0.2 0.21428571 0.22857143 0.24285714 0.25714286 0.27142857 0.28571429 0.3 0.31428571 0.32857143 0.34285714 0.35714286 0.37142857 0.38571429 0.4 0.41428571 0.42857143 0.44285714 0.45714286 0.47142857 0.48571429 0.5 0.51428571 0.52857143 0.54285714 0.55714286 0.57142857 0.58571429 0.6 0.61428571 0.62857143 0.64285714 0.65714286 0.67142857 0.68571429 0.7 0.71428571 0.72857143 0.74285714 0.75714286 0.77142857 0.78571429 0.8 0.81428571 0.82857143 0.84285714 0.85714286 0.87142857 0.88571429 0.9 0.91428571 0.92857143 0.94285714 0.95714286 0.97142857 0.98571429 1 1 1 1 1 1
  arc A0 (8.1516, -0.3707) -> (8.1516, 0.3707) centre (0, 0) ccw
  line L0 (5.8182, -0.6584) -> (6.8689, -0.776)
  line L1 (5.8182, 0.6584) -> (6.8689, 0.776)
  line L2 (5.8182, -0.6584) -> (5.8182, 0.6584)
  point P0 (6.9585, -0.7764)
  point P1 (7.049, -0.7688)
  point P2 (7.14, -0.7557)
  point P3 (7.2314, -0.738)
  point P4 (7.3231, -0.7162)
  point P5 (7.4151, -0.6907)
  point P6 (7.5072, -0.6617)
  point P7 (7.5994, -0.6293)
  point P8 (7.6916, -0.5938)
  point P9 (7.7838, -0.5551)
  point P10 (7.876, -0.5133)
  point P11 (7.968, -0.4687)
  point P12 (8.0599, -0.4211)
  point P13 (6.9585, 0.7764)
  point P14 (7.049, 0.7688)
  point P15 (7.14, 0.7557)
  point P16 (7.2314, 0.738)
  point P17 (7.3231, 0.7162)
  point P18 (7.4151, 0.6907)
  point P19 (7.5072, 0.6617)
  point P20 (7.5994, 0.6293)
  point P21 (7.6916, 0.5938)
  point P22 (7.7838, 0.5551)
  point P23 (7.876, 0.5133)
  point P24 (7.968, 0.4687)
  point P25 (8.0599, 0.4211)
extrude "Extrude2''''" add sketch "Sketch2 (3)" along normal blind 6.5 bodies 34 in component "Spur Gear (14 teeth) (1)"
fillet "Fillet1''" radius 0.6 2 edges at (5.828, -0.6595, 3.25) (5.828, 0.6595, 3.25) on bodies 34 in component "Spur Gear (14 teeth) (1)"
pattern_circular "C-Pattern1'" count 14 over 360 about axis through (0, 0, 0) along (0, 0, 1) of "Extrude2''''", "Fillet1''" in component "Spur Gear (14 teeth) (1)"
sketch "Sketch3 (2)" plane through (0, 0, 0) normal (0, 0, 1) x (1, 0, 0) in component "Spur Gear (14 teeth) (1)"
  circle A0 centre (0, 0) radius 7.14 construction
cylinder "CylinderPrimitive1'" cut diameter 5.7 height -3.2 placed x (1, 0, 0) y (0, 1, 0) z (0, 0, 1) at (0, 0, 6.5) bodies 34 in component "Spur Gear (14 teeth) (1)"
cylinder "CylinderPrimitive2'" cut diameter 6.2 height -2.4 placed x (0, 1, 0) y (1, 0, 0) z (0, 0, -1) at (0, 0, 0) bodies 34 in component "Spur Gear (14 teeth) (1)"
sketch "Sketch1 (6)" plane through (0, 0, 0) normal (0, 0, 1) x (1, 0, 0) in component "JawRing"
  line L0 (-28, 16) -> (28, 16)
  line L1 (28, 16) -> (28, 8.75)
  line L2 (28, 8.75) -> (-28, 8.75)
  line L3 (-28, 8.75) -> (-28, 16)
  line L4 (11.5, 16) -> (28, 16)
  line L5 (28, 16) -> (28, -8)
  line L6 (28, -8) -> (11.5, -8)
  line L7 (11.5, -8) -> (11.5, 16)
  line L8 (11.5, -5) -> (24.8331, -5)
  line L9 (24.8331, -5) -> (24.8331, 5)
  line L10 (24.8331, 5) -> (11.5, 5)
  line L11 (11.5, 5) -> (11.5, -5)
  circle A0 centre (20.4076, 12.375) radius 1.6
  circle A1 centre (-20.3901, 12.3735) radius 1.6
  line L12 (-16.3901, 8.8735) -> (-24.3901, 8.8735)
  line L13 (-24.3901, 8.8735) -> (-24.3901, 15.8735)
  line L14 (-24.3901, 15.8735) -> (-16.3901, 15.8735)
  line L15 (-16.3901, 15.8735) -> (-16.3901, 8.8735)
  line L16 (-16.3901, 8.8735) -> (-24.3901, 15.8735) construction
  line L17 (-24.3901, 8.8735) -> (-16.3901, 15.8735) construction
  line L18 (-18.7157, 9.4735) -> (-17.0414, 12.3735)
  line L19 (-17.0414, 12.3735) -> (-18.7157, 15.2735)
  line L20 (-18.7157, 15.2735) -> (-22.0644, 15.2735)
  line L21 (-22.0644, 15.2735) -> (-23.7387, 12.3735)
  line L22 (-23.7387, 12.3735) -> (-22.0644, 9.4735)
  line L23 (-22.0644, 9.4735) -> (-18.7157, 9.4735)
  line L24 (24.4076, 8.875) -> (16.4076, 8.875)
  line L25 (16.4076, 8.875) -> (16.4076, 15.875)
  line L26 (16.4076, 15.875) -> (24.4076, 15.875)
  line L27 (24.4076, 15.875) -> (24.4076, 8.875)
  line L28 (24.4076, 8.875) -> (16.4076, 15.875) construction
  line L29 (16.4076, 8.875) -> (24.4076, 15.875) construction
  line L30 (22.0819, 9.475) -> (23.7562, 12.375)
  line L31 (23.7562, 12.375) -> (22.0819, 15.275)
  line L32 (22.0819, 15.275) -> (18.7333, 15.275)
  line L33 (18.7333, 15.275) -> (17.0589, 12.375)
  line L34 (17.0589, 12.375) -> (18.7333, 9.475)
  line L35 (18.7333, 9.475) -> (22.0819, 9.475)
  point P0 (-28, 16)
  point P1 (28, 8.75)
  point P2 (-20.3901, 12.3735)
  point P3 (-20.3901, 12.3735)
  point P4 (20.4076, 12.375)
  point P5 (20.4076, 12.375)
  dimension "d99_1" = 3.2
  dimension "d100_1" = 3.2
  dimension "d115_1" = 8
  dimension "d116_1" = 7
  dimension "d117_1" = 8
  dimension "d118_1" = 7
  dimension "d153_1" = 39.5
  dimension "d154_1" = 16.5
  constraint horizontal L0
  constraint vertical L1
  constraint horizontal L2
  constraint vertical L3
  constraint coincident P1 L1.end
  constraint coincident P0 L0.start
  constraint horizontal L4
  constraint vertical L5
  constraint horizontal L6
  constraint vertical L7
  constraint coincident L0 L4.start
  constraint horizontal L8
  constraint vertical L9
  constraint horizontal L10
  constraint vertical L11
  constraint coincident L7 L8.start
  constraint perpendicular L12 L13
  constraint parallel L12 L14
  constraint parallel L13 L15
  constraint horizontal L12
  constraint coincident L16 P3
  constraint coincident L17 P3
  constraint coincident P3 P2
  constraint perpendicular L24 L25
  constraint parallel L24 L26
  constraint parallel L25 L27
  constraint horizontal L24
  constraint coincident L28 P5
  constraint coincident L29 P5
  constraint coincident P5 P4
  measures "d99_1" diameter of A0
  measures "d100_1" diameter of A1
  measures "d115_1" distance of L13.end L14.end
  measures "d116_1" distance of L12.end L13.end
  measures "d117_1" distance of L25.end L26.end
  measures "d118_1" distance of L24.end L25.end
  measures "d153_1" distance of L3 L7
  measures "d154_1" horizontal distance of L5.end L6.end
extrude "Extrude1'''''" add sketch "Sketch1 (6)" along normal blind 3 separate body contours L0 L2 L3 L7 | L0 L1 L2 L4 L5 L7 | L2 L5 L6 L7 L8 L9 L10 | L7 L8 L9 L10 L11 | L12 L13 L14 L15 | L18 L19 L20 L21 L22 L23 | L24 L25 L26 L27 | L30 L31 L32 L33 L34 L35 makes body 35 in component "JawRing"
extrude "Extrude2'''''" add sketch "Sketch1 (6)" along normal blind 6 separate body contours L2 L5 L6 L7 L8 L9 L10 | L7 L8 L9 L10 L11 makes body 36 in component "JawRing"
chamfer "Chamfer1''" distance 3 angle 45 1 edges at (19.75, -8, 6) on bodies 36 in component "JawRing"
chamfer "Chamfer2'" distance 3 angle 45 1 edges at (28, 1.875, 6) on bodies 36 in component "JawRing"
chamfer "Chamfer3'" distance 3.75 angle 45 1 edges at (18.25, 8.75, 6) on bodies 36 in component "JawRing"
extrude "Extrude3'''" add sketch "Sketch1 (6)" along normal blind 45 contours L7 L8 L9 L10 L11 bodies 35 36 in component "JawRing"
chamfer "Chamfer4'" distance 8 distance2 39 1 edges at (24.8331, 0, 45) measured on face at (15.9444, -1.6667, 45) on bodies 35 in component "JawRing"
fillet "Fillet1'''" radius 5 2 edges at (20.8331, -5, 25.5) (20.8331, 5, 25.5) on bodies 35 in component "JawRing"
extrude "Extrude4'''" add sketch "Sketch1 (6)" along normal blind 6 separate body contours L12 L13 L14 L15 | L24 L25 L26 L27 makes body 37 at (-19.0567, 8.8735, 2) makes body 38 at (21.7409, 8.875, 2) in component "JawRing"
fillet "Fillet3''" radius 2 4 edges at (-24.3901, 8.8735, 3) (-16.3901, 8.8735, 3) (-16.3901, 15.8735, 3) (-24.3901, 15.8735, 3) on bodies 37 in component "JawRing"
fillet "Fillet4'" radius 2 4 edges at (16.4076, 15.875, 3) (24.4076, 15.875, 3) (24.4076, 8.875, 3) (16.4076, 8.875, 3) on bodies 38 in component "JawRing"
fillet "Fillet5'" radius 1 5 edges at (28, -8, 1.5) (11.5, -8, 1.5) (28, 16, 1.5) (-28, 16, 1.5) (-28, 8.75, 1.5) on bodies 35 in component "JawRing"
box "BoxPrimitive1'''" add length 7 width 6 height 2 placed x (0, 1, 0) y (-1, 0, 0) z (0, 0, 1) at (37, -1, 0) separate body makes body 39 in component "JawRing"
chamfer "Chamfer5'" distance 3 distance2 2 1 edges at (31, 2.5, 2) measured on face at (33, 1.3333, 2) on bodies 39 in component "JawRing"
move_body "Move1''''" bodies 39 to x (1, 0, 0) y (0, 1, 0) z (0, 0, 1) at (-6, 0, 0) in component "JawRing"
combine "Combine1'" operation cut target body 35 tool bodies 39 in component "JawRing"
fillet "Fillet6'" radius 4 4 edges at (11.6145, 5, 45) (15.3381, 3.5355, 45) (15.3381, -3.5355, 45) (11.6145, -5, 45) on bodies 35 in component "JawRing"
box "BoxPrimitive2''" add length 12 width 20 height 50 placed x (0, -1, 0) y (1, 0, 0) z (0, 0, 1) at (30, 6, 0) separate body makes body 40 in component "JawRing"
move_body "Move2'''" bodies 40 to x (1, 0, 0) y (0, 1, 0) z (0, 0, 1) at (0, 0, 6) in component "JawRing"
move_body "Move3''" bodies 40 to x (1, 0, 0) y (0, 1, 0) z (0, 0, 1) at (-19.9434, 0, 0) in component "JawRing"
combine "Combine2" operation cut target body 35 tool bodies 40 in component "JawRing"
extrude "Extrude5''" add 1 faces at (14.2435, 1.6667, 6) along direction (0, 0, 1) blind 6 on bodies 35 bodies 35 in component "JawRing"
torus "TorusPrimitive1" add centre line diameter 32 section diameter 6 placed x (0, 1, 0) y (0, 0, 1) z (1, 0, 0) at (0, 0, 30) separate body makes body 41 in component "JawRing"
move_body "Move4''" bodies 41 to x (1, 0, 0) y (0, 1, 0) z (0, 0, 1) at (20, 0, 0) in component "JawRing"
move_body "Move5''" bodies 41 to x (1, 0, 0) y (0, 1, 0) z (0, 0, 1) at (0, 0, -4) in component "JawRing"
fillet "Fillet7" radius 2.5 1 edges at (25, 0, 12) on bodies 35 in component "JawRing"
chamfer "Chamfer6" distance 4 angle 45 1 edges at (11.5, 0, 12) on bodies 35 in component "JawRing"
fillet "Fillet8" radius 5.305 1 edges at (15.5, 0, 12) on bodies 35 in component "JawRing"
fillet "Fillet9" radius 9.355 1 edges at (11.5, 0, 8) on bodies 35 in component "JawRing"
fillet "Fillet1''''" [suppressed] in component "Rack"
component "Rack" placed x (1, 0, 0) y (0, 1, 0) z (0, 0, 1) at (0, 0, 0)
component "Base" placed x (1, 0, 0) y (0, 1, 0) z (0, 0, 1) at (0, 0, 0)
component "Jaw" placed x (1, 0, 0) y (0, 1, 0) z (0, 0, 1) at (0, 0, 0)
component "Spur Gear (14 teeth) (1)" placed x (1, 0, 0) y (0, 1, 0) z (0, 0, 1) at (0, 0, 0)
hidden bodies 2
